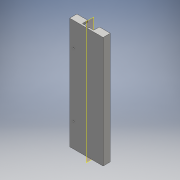
# Autodesk Inventor part: Base
Saved by Autodesk Inventor 2016 (Build 200138000, 138)
## iProperties
Created: 2015-08-31
Part Number: Base
Material: Generic
Document SubType Name: Modeling
Designer: amatiasq
Density: 1 g/cm^3
Appearance: Default
Author: amatiasq
Autodesk Inventor part; units mm, degrees
ref_plane "YZ Plane" through (0, 0, 0) normal (1, 0, 0) x (0, 1, 0)
ref_plane "XZ Plane" through (0, 0, 0) normal (0, 1, 0) x (-1, 0, 0)
ref_plane "XY Plane" through (0, 0, 0) normal (0, 0, 1) x (1, 0, 0)
sketch "Sketch1" plane through (0, 0, 0) normal (0, 1, 0) x (-1, 0, 0)
  line L0 (0, 0) -> (-60, 0)
  line L1 (-60, 0) -> (-60, -200)
  line L2 (-60, -200) -> (0, -200)
  line L3 (0, -200) -> (0, 0)
  dimension "d0" = 60
  dimension "d1" = 200
  constraints: 8 end point, 2 parallel, 1 horizontal, 1 perpendicular
  measures "d0" distance of L2.end L1.end
  measures "d1" distance of L1.end L0.end
extrude "Base" add sketch "Sketch1" along normal blind 3
sketch "Sketch4" plane through (0, 3, 0) normal (0, 1, 0) x (1, 0, 0)
  line L0 (0, 0) -> (60, 0) projected
  line L1 (60, 0) -> (60, 200) projected
  line L2 (60, 200) -> (0, 200) projected
  line L3 (0, 200) -> (0, 0) projected
  line L4 (3, 3) -> (57, 3)
  line L5 (57, 3) -> (57, 197)
  line L6 (57, 197) -> (3, 197)
  line L7 (3, 197) -> (3, 3)
  line L8 (19.7, 0) -> (40.3, 0)
  line L9 (40.3, 0) -> (40.3, 3)
  line L10 (40.3, 3) -> (19.7, 3)
  line L11 (19.7, 3) -> (19.7, 0)
  point P0 (30, 0)
  point P1 (30, 3)
  dimension "d6" = 3
  dimension "d7" = 20.6
  constraints: 16 end point, 4 midpoint, 2 parallel, 1 horizontal, 1 perpendicular, 3 other
  measures "d6" distance between parallel lines of L3 L7
  measures "d7" distance between parallel lines of L9 L11
extrude "Paredes" add sketch "Sketch4" along normal blind 10 contours L3 L2 L1 L0 L9 L4 L5 L6 L7 L11
sketch "Sketch5" plane through (0, 3, 0) normal (0, 1, 0) x (1, 0, 0)
  line L0 (27.5, 0) -> (32.5, 0)
  line L1 (32.5, 0) -> (32.5, 197)
  line L2 (32.5, 197) -> (27.5, 197)
  line L3 (27.5, 197) -> (27.5, 0)
  line L4 (19.7, 0) -> (40.3, 0) projected
  line L5 (57, 197) -> (3, 197) projected
  point P0 (0, 0)
  point P1 (30, 0)
  point P2 (30, 197)
  dimension "d10" = 5
  constraints: 8 end point, 4 midpoint, 2 parallel, 1 horizontal, 1 perpendicular
  measures "d10" distance between parallel lines of L1 L3
extrude "Canal" cut sketch "Sketch5" against normal blind 1.5
sketch "Sketch6" plane through (0, 3, 0) normal (0, 1, 0) x (1, 0, 0)
  line L0 (7, 3.0083) -> (7, 197)
  line L1 (27.5, 197) -> (3, 197) projected
  line L2 (3, 197) -> (3, 3) projected
  line L3 (3, 3) -> (19.7, 3) projected
  point P0 (0, 0)
  point P1 (7, 43)
  point P2 (7, 157)
  dimension "d13" = 4
  dimension "d14" = 40
  dimension "d15" = 40
  constraints: 3 point on line, 2 end point, 1 vertical
  measures "d13" distance between parallel lines of L0 L2
  measures "d14" distance from line of L3 point (7, 43)
  measures "d15" distance from line of L1 point (7, 157)
hole "Agujeros" at (7, 3, -43) at (7, 3, -157) direction (0, -1, 0) diameter 2 end through all
ref_plane "Mitad" through (30, 3, -3) normal (1, 0, 0) x (0, 0, -1)
sketch "Sketch9" plane through (0, 3, 0) normal (0, 1, 0) x (1, 0, 0)
  line L0 (9.4, 50) -> (14.4, 50)
  line L1 (14.4, 50) -> (14.4, 150)
  line L2 (14.4, 150) -> (9.4, 150)
  line L3 (9.4, 150) -> (9.4, 50)
  line L4 (30, 240) -> (30, -40) projected
  line L5 (3, 197) -> (3, 3) projected
  line L6 (3, 100) -> (57, 100)
  line L7 (57, 197) -> (57, 3) projected
  point P0 (0, 0)
  point P1 (14.4, 100)
  dimension "d23" = 15.6
  dimension "d24" = 100
  dimension "d25" = 5
  constraints: 10 end point, 3 midpoint, 2 parallel, 1 horizontal, 1 perpendicular, 1 point on line
  measures "d23" distance between parallel lines of L1 L4
  measures "d24" distance between parallel lines of L2 L0
  measures "d25" distance between parallel lines of L3 L1
extrude "Soporte base" add sketch "Sketch9" along normal blind 4
chamfer "Chaflán soporte" distance 2.5 angle 45 2 edges at (14.4, 5, -50) (14.4, 5, -150)
sketch "Sketch10" plane through (0, 7, 0) normal (0, 1, 0) x (1, 0, 0)
  line L0 (9.4, 90) -> (14.4, 90)
  line L1 (14.4, 90) -> (14.4, 110)
  line L2 (14.4, 110) -> (9.4, 110)
  line L3 (9.4, 110) -> (9.4, 90)
  line L4 (9.4, 150) -> (9.4, 50) projected
  line L5 (14.4, 52.5) -> (14.4, 147.5) projected
  point P0 (0, 0)
  point P1 (9.4, 100)
  point P2 (14.4, 100)
  dimension "d31" = 20
  constraints: 8 end point, 4 midpoint, 2 parallel, 1 horizontal, 1 perpendicular
  measures "d31" distance between parallel lines of L2 L0
extrude "Soporte tope" add sketch "Sketch10" along normal blind 5
mirror "Segundo soporte" about plane through (30, 3, -3) normal (1, 0, 0) of "Soporte base", "Chaflán soporte", "Soporte tope"
equation "\"d0\" = base_ancho"
equation "\"d1\" = base_largo"
equation "\"d2\" = base_alto"
equation "\"d6\" = muros_grosor"
equation "\"d7\" = hoja_ancho + 2 * margen"
equation "\"d8\" = muros_alto"
equation "\"d10\" = rail_grosor"
equation "\"d11\" = rail_alto"
equation "\"d21\" = d14"
equation "\"d23\" = 0.5 * hoja_ancho_total + 2 * margen"
equation "\"d24\" = deslizador_soporte_largo"
equation "\"d25\" = deslizador_soporte_ancho"
equation "\"d26\" = deslizador_soporte_alto"
equation "\"d28\" = 0.5 * deslizador_soporte_ancho"
equation "\"d31\" = deslizador_tope_largo"
equation "\"d32\" = deslizador_tope_alto"
equation "\"margen\" = 0.3"
equation "\"hoja_stop_largo\" = 5"
equation "\"hoja_stop_saliente\" = 5"
equation "\"hoja_stop_posicion\" = 5"
equation "\"hoja_alto\" = 3"
equation "\"rail_grosor\" = 5"
equation "\"base_alto\" = 3"
equation "\"base_ancho\" = 60"
equation "\"base_largo\" = 200"
equation "\"muros_alto\" = 10"
equation "\"muros_grosor\" = 3"
equation "\"rail_alto\" = 1.5"
equation "\"hoja_stop_biselado\" = 2"
equation "\"hoja_cola_biselado\" = 1"
equation "\"hoja_filo_biselado\" = 0.5"
equation "\"deslizador_soporte_alto\" = 4"
equation "\"deslizador_soporte_ancho\" = 5"
equation "\"deslizador_tope_alto\" = 5"
equation "\"deslizador_soporte_largo\" = 100"
equation "\"deslizador_tope_largo\" = 20"
equation "\"deslizador_alto\" = 3"
equation "\"tirador_agarre_largo\" = 3"
equation "\"deslizador_saliente\" = 5"
equation "\"deslizador_largo\" = 154"
equation "\"deslizador_interruptor_largo\" = 5"
equation "\"deslizador_interruptor_ancho\" = 7"
equation "\"hoja_ancho\" = 20"
equation "\"hoja_ancho_total\" = 30"
body "Solid1"
